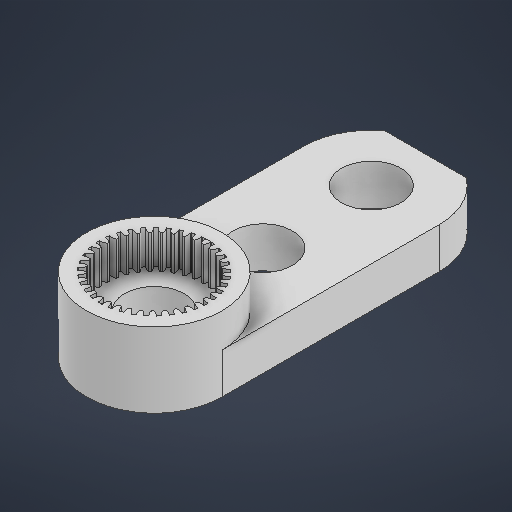
# Autodesk Inventor part: digital servo cap
Saved by Autodesk Inventor 2026.1 (Build 301233020, 233B)
## iProperties
Created: 2025-11-05
Part Number: digital servo cap
Material: Generic
Document SubType Name: Modeling
Designer: Asus
Density: 1 g/cm^3
Appearance: Default
Author: Asus
Autodesk Inventor part; units mm, degrees
ref_plane "YZ Plane" through (0, 0, 0) normal (1, 0, 0) x (0, 1, 0)
ref_plane "XZ Plane" through (0, 0, 0) normal (0, 1, 0) x (-1, 0, 0)
ref_plane "XY Plane" through (0, 0, 0) normal (0, 0, 1) x (1, 0, 0)
sketch "Sketch1" plane through (0, 0, 0) normal (0, 1, 0) x (-1, 0, 0)
  line L0 (0, 0) -> (0, -16) construction
  line L1 (-5, 0) -> (-5, -16)
  line L2 (5, -16) -> (5, 0)
  arc A0 (5, 0) -> (-5, 0) centre (0, 0) ccw
  circle A1 centre (0, 0) radius 2.2
  circle A2 centre (0, -16) radius 2.2
  line L3 (0, -16) -> (0, -20)
  line L4 (0, -20) -> (3, -20)
  line L5 (3, -20) -> (-3, -20)
  arc A3 (-5, -16) -> (-3, -20) centre (0, -16) ccw
  arc A4 (3, -20) -> (5, -16) centre (0, -16) ccw
  circle A5 centre (0, -8) radius 2.2
  dimension "d0" = 16
  dimension "d2" = 4.4
  dimension "d3" = 4.4
  dimension "d4" = 4
  dimension "d5" = 4.4
  constraints: 14 end point, 6 centre point, 6 point on circle, 4 tangent, 3 coincident, 2 vertical, 1 midpoint, 1 parallel, 1 perpendicular
  measures "d0" distance of L0.start L0.end
  measures "d2" diameter of A1
  measures "d3" diameter of A2
  measures "d4" distance of L3.start L3.end
  measures "d5" diameter of A5
extrude "Extrusion1" add sketch "Sketch1" along normal blind 3
sketch "Sketch2" plane through (0, 3, 0) normal (0, 1, 0) x (1, 0, 0)
  circle A0 centre (0, 0) radius 4
  circle A1 centre (0, 0) radius 5
  dimension "d8" = 8
  constraints: 2 centre point, 2 coincident
  measures "d8" diameter of A0
extrude "Extrusion2" add sketch "Sketch2" along normal blind 2.5
sketch "Sketch3" plane through (0, 5.5, 0) normal (0, 1, 0) x (1, 0, 0)
  circle A0 centre (0, 0) radius 4
  circle A1 centre (0, 0) radius 4 projected
  line L0 (0, 4.0912) -> (0, 3.5243) construction
  line L1 (-0.2, 3.995) -> (0.2, 3.995)
  circle A2 centre (0, 0) radius 4 projected
  line L2 (0, 3.545) -> (0.075, 3.545)
  line L3 (0, 3.545) -> (-0.075, 3.545)
  arc A3 (-0.1998, 3.9692) -> (-0.075, 3.545) centre (0.65, 3.9887) ccw
  arc A4 (0.075, 3.545) -> (0.1998, 3.9692) centre (-0.65, 3.9887) ccw
  arc A5 (0.2262, 3.9936) -> (0.1998, 3.9692) centre (0.2248, 3.9686) ccw
  arc A6 (-0.1998, 3.9692) -> (-0.2262, 3.9936) centre (-0.2248, 3.9686) ccw
  line L4 (-0.5991, 3.494) -> (-0.673, 3.4813)
  line L5 (-0.5991, 3.494) -> (-0.5252, 3.5067)
  arc A7 (-0.5252, 3.5067) -> (-0.4739, 3.9459) centre (-1.3147, 3.8215) ccw
  arc A8 (-0.8677, 3.8784) -> (-0.673, 3.4813) centre (-0.0335, 4.0412) ccw
  arc A9 (-0.8677, 3.8784) -> (-0.8979, 3.8979) centre (-0.8923, 3.8736) ccw
  arc A10 (-0.452, 3.9744) -> (-0.4739, 3.9459) centre (-0.4491, 3.9495) ccw
  line L6 (-1.181, 3.3425) -> (-1.2517, 3.3175)
  line L7 (-1.181, 3.3425) -> (-1.1103, 3.3675)
  arc A11 (-1.1103, 3.3675) -> (-1.1339, 3.809) centre (-1.9417, 3.5444) ccw
  arc A12 (-1.5107, 3.6759) -> (-1.2517, 3.3175) centre (-0.716, 3.9774) ccw
  arc A13 (-1.5107, 3.6759) -> (-1.5437, 3.6901) centre (-1.5341, 3.6671) ccw
  arc A14 (-1.1171, 3.8408) -> (-1.1339, 3.809) centre (-1.1102, 3.8168) ccw
  line L8 (-1.7289, 3.0948) -> (-1.7944, 3.0583)
  line L9 (-1.7289, 3.0948) -> (-1.6634, 3.1314)
  arc A15 (-1.6634, 3.1314) -> (-1.7613, 3.5626) centre (-2.5127, 3.1652) ccw
  arc A16 (-2.1102, 3.3677) -> (-1.7944, 3.0583) centre (-1.3778, 3.7992) ccw
  arc A17 (-2.1102, 3.3677) -> (-2.1451, 3.3761) centre (-2.1317, 3.355) ccw
  arc A18 (-1.7502, 3.5968) -> (-1.7613, 3.5626) centre (-1.7392, 3.5743) ccw
  line L10 (-2.227, 2.7581) -> (-2.2854, 2.711)
  line L11 (-2.227, 2.7581) -> (-2.1687, 2.8053)
  arc A19 (-2.1687, 2.8053) -> (-2.3381, 3.2137) centre (-3.0115, 2.6951) ccw
  arc A20 (-2.649, 2.9627) -> (-2.2854, 2.711) centre (-2.0001, 3.5117) ccw
  arc A21 (-2.649, 2.9627) -> (-2.6849, 2.9651) centre (-2.6681, 2.9465) ccw
  arc A22 (-2.3329, 3.2493) -> (-2.3381, 3.2137) centre (-2.3183, 3.229) ccw
  line L12 (-2.6611, 2.3421) -> (-2.7107, 2.2858)
  line L13 (-2.6611, 2.3421) -> (-2.6116, 2.3984)
  arc A23 (-2.6116, 2.3984) -> (-2.8476, 2.7723) centre (-3.4237, 2.1473) ccw
  arc A24 (-3.1116, 2.4724) -> (-2.7107, 2.2858) centre (-2.5648, 3.1232) ccw
  arc A25 (-3.1116, 2.4724) -> (-3.1473, 2.4687) centre (-3.1277, 2.4532) ccw
  arc A26 (-2.8484, 2.8083) -> (-2.8476, 2.7723) centre (-2.8306, 2.7907) ccw
  line L14 (-3.0187, 1.8587) -> (-3.058, 1.7948)
  line L15 (-3.0187, 1.8587) -> (-2.9793, 1.9225)
  arc A27 (-2.9793, 1.9225) -> (-3.2751, 2.2512) centre (-3.7373, 1.5379) ccw
  arc A28 (-3.4847, 1.911) -> (-3.058, 1.7948) centre (-3.0557, 2.6448) ccw
  arc A29 (-3.4847, 1.911) -> (-3.5193, 1.9013) centre (-3.4973, 1.8894) ccw
  arc A30 (-3.2821, 2.2865) -> (-3.2751, 2.2512) centre (-3.2616, 2.2722) ccw
  line L16 (-3.2894, 1.3218) -> (-3.3173, 1.2522)
  line L17 (-3.2894, 1.3218) -> (-3.2614, 1.3914)
  arc A31 (-3.2614, 1.3914) -> (-3.6085, 1.6653) centre (-3.9435, 0.8841) ccw
  arc A32 (-3.7575, 1.2946) -> (-3.3173, 1.2522) centre (-3.4588, 2.0903) ccw
  arc A33 (-3.7575, 1.2946) -> (-3.79, 1.2791) centre (-3.7663, 1.2712) ccw
  arc A34 (-3.6213, 1.6989) -> (-3.6085, 1.6653) centre (-3.5986, 1.6883) ccw
  line L18 (-3.4654, 0.7469) -> (-3.4812, 0.6735)
  line L19 (-3.4654, 0.7469) -> (-3.4496, 0.8202)
  arc A35 (-3.4496, 0.8202) -> (-3.838, 1.0315) centre (-4.0362, 0.205) ccw
  arc A36 (-3.9222, 0.6409) -> (-3.4812, 0.6735) centre (-3.7623, 1.4757) ccw
  arc A37 (-3.9222, 0.6409) -> (-3.9516, 0.6202) centre (-3.9269, 0.6164) ccw
  arc A38 (-3.8563, 1.0625) -> (-3.838, 1.0315) centre (-3.8322, 1.0559) ccw
  line L20 (-3.5418, 0.1505) -> (-3.545, 0.0755)
  line L21 (-3.5418, 0.1505) -> (-3.5386, 0.2254)
  arc A39 (-3.5386, 0.2254) -> (-3.9572, 0.3681) centre (-4.0127, -0.4801) ccw
  arc A40 (-3.9741, -0.0312) -> (-3.545, 0.0755) centre (-3.9576, 0.8187) ccw
  arc A41 (-3.9741, -0.0312) -> (-3.9996, -0.0565) centre (-3.9746, -0.0562) ccw
  arc A42 (-3.9804, 0.3955) -> (-3.9572, 0.3681) centre (-3.9555, 0.393) ccw
  line L22 (-3.5163, -0.4503) -> (-3.5068, -0.5247)
  line L23 (-3.5163, -0.4503) -> (-3.5258, -0.3759)
  arc A43 (-3.5258, -0.3759) -> (-3.9624, -0.306) centre (-3.8739, -1.1514) ccw
  arc A44 (-3.9117, -0.7023) -> (-3.5068, -0.5247) centre (-4.039, 0.1381) ccw
  arc A45 (-3.9117, -0.7023) -> (-3.9325, -0.7316) centre (-3.9079, -0.7271) ccw
  arc A46 (-3.99, -0.2829) -> (-3.9624, -0.306) centre (-3.965, -0.2811) ccw
  line L24 (-3.3896, -1.0381) -> (-3.3676, -1.1098)
  line L25 (-3.3896, -1.0381) -> (-3.4116, -0.9663)
  arc A47 (-3.4116, -0.9663) -> (-3.8537, -0.9712) centre (-3.6236, -1.7895) ccw
  arc A48 (-3.7367, -1.3533) -> (-3.3676, -1.1098) centre (-4.0042, -0.5465) ccw
  arc A49 (-3.7367, -1.3533) -> (-3.7523, -1.3857) centre (-3.7289, -1.377) ccw
  arc A50 (-3.8848, -0.9531) -> (-3.8537, -0.9712) centre (-3.8605, -0.9472) ccw
  line L26 (-3.1654, -1.596) -> (-3.1317, -1.6629)
  line L27 (-3.1654, -1.596) -> (-3.1992, -1.529)
  arc A51 (-3.1992, -1.529) -> (-3.6342, -1.6085) centre (-3.269, -2.3761) ccw
  arc A52 (-3.4543, -1.9654) -> (-3.1317, -1.6629) centre (-3.8543, -1.2154) ccw
  arc A53 (-3.4543, -1.9654) -> (-3.4641, -1.9999) centre (-3.4425, -1.9874) ccw
  arc A54 (-3.6678, -1.5959) -> (-3.6342, -1.6085) centre (-3.6449, -1.586) ccw
  line L28 (-2.8502, -2.108) -> (-2.8056, -2.1683)
  line L29 (-2.8502, -2.108) -> (-2.8948, -2.0477)
  arc A55 (-2.8948, -2.0477) -> (-3.31, -2.1996) centre (-2.8204, -2.8944) ccw
  arc A56 (-3.0724, -2.5209) -> (-2.8056, -2.1683) centre (-3.5934, -1.8493) ccw
  arc A57 (-3.0724, -2.5209) -> (-3.0763, -2.5566) centre (-3.0571, -2.5406) ccw
  arc A58 (-3.3454, -2.1929) -> (-3.31, -2.1996) centre (-3.3244, -2.1792) ccw
  line L30 (-2.4529, -2.5593) -> (-2.3988, -2.6112)
  line L31 (-2.4529, -2.5593) -> (-2.5071, -2.5074)
  arc A59 (-2.5071, -2.5074) -> (-2.8907, -2.7273) centre (-2.2907, -3.3294) ccw
  arc A60 (-2.6022, -3.0038) -> (-2.3988, -2.6112) centre (-3.2292, -2.43) ccw
  arc A61 (-2.6022, -3.0038) -> (-2.6, -3.0397) centre (-2.5838, -3.0207) ccw
  arc A62 (-2.9266, -2.7267) -> (-2.8907, -2.7273) centre (-2.9083, -2.7096) ccw
  line L32 (-1.9851, -2.9371) -> (-1.923, -2.9791)
  line L33 (-1.9851, -2.9371) -> (-2.0472, -2.8951)
  arc A63 (-2.0472, -2.8951) -> (-2.3882, -3.1766) centre (-1.6951, -3.6687) ccw
  arc A64 (-2.0571, -3.4004) -> (-1.923, -2.9791) centre (-2.7721, -2.9407) ccw
  arc A65 (-2.0571, -3.4004) -> (-2.0489, -3.4354) centre (-2.0361, -3.4139) ccw
  arc A66 (-2.4237, -3.1821) -> (-2.3882, -3.1766) centre (-2.4086, -3.1622) ccw
  line L34 (-1.4602, -3.2303) -> (-1.3918, -3.2612)
  line L35 (-1.4602, -3.2303) -> (-1.5285, -3.1994)
  arc A67 (-1.5285, -3.1994) -> (-1.817, -3.5346) centre (-1.0507, -3.9024) ccw
  arc A68 (-1.4529, -3.6992) -> (-1.3918, -3.2612) centre (-2.2352, -3.3669) ccw
  arc A69 (-1.4529, -3.6992) -> (-1.4388, -3.7323) centre (-1.4299, -3.7089) ccw
  arc A70 (-1.8511, -3.5459) -> (-1.817, -3.5346) centre (-1.8395, -3.5237) ccw
  line L36 (-0.8933, -3.4306) -> (-0.8207, -3.4495)
  line L37 (-0.8933, -3.4306) -> (-0.9658, -3.4117)
  arc A71 (-0.9658, -3.4117) -> (-1.1935, -3.7908) centre (-0.3761, -4.0238) ccw
  arc A72 (-0.8068, -3.8915) -> (-0.8207, -3.4495) centre (-1.6341, -3.6963) ccw
  arc A73 (-0.8068, -3.8915) -> (-0.7874, -3.9217) centre (-0.7825, -3.8972) ccw
  arc A74 (-1.2252, -3.8077) -> (-1.1935, -3.7908) centre (-1.2175, -3.7839) ccw
  line L38 (-0.3006, -3.5322) -> (-0.2259, -3.5386)
  line L39 (-0.3006, -3.5322) -> (-0.3754, -3.5259)
  arc A75 (-0.3754, -3.5259) -> (-0.5357, -3.938) centre (0.3094, -4.0295) ccw
  arc A76 (-0.1375, -3.9719) -> (-0.2259, -3.5386) centre (-0.9859, -3.9192) ccw
  arc A77 (-0.1375, -3.9719) -> (-0.1133, -3.9984) centre (-0.1126, -3.9734) ccw
  arc A78 (-0.5641, -3.96) -> (-0.5357, -3.938) centre (-0.5605, -3.9353) ccw
  line L40 (0.3006, -3.5322) -> (0.3754, -3.5259)
  line L41 (0.3006, -3.5322) -> (0.2259, -3.5386)
  arc A79 (0.2259, -3.5386) -> (0.1375, -3.9719) centre (0.9859, -3.9192) ccw
  arc A80 (0.5357, -3.938) -> (0.3754, -3.5259) centre (-0.3094, -4.0295) ccw
  arc A81 (0.5357, -3.938) -> (0.5641, -3.96) centre (0.5605, -3.9353) ccw
  arc A82 (0.1133, -3.9984) -> (0.1375, -3.9719) centre (0.1126, -3.9734) ccw
  line L42 (0.8933, -3.4306) -> (0.9658, -3.4117)
  line L43 (0.8933, -3.4306) -> (0.8207, -3.4495)
  arc A83 (0.8207, -3.4495) -> (0.8068, -3.8915) centre (1.6341, -3.6963) ccw
  arc A84 (1.1935, -3.7908) -> (0.9658, -3.4117) centre (0.3761, -4.0238) ccw
  arc A85 (1.1935, -3.7908) -> (1.2252, -3.8077) centre (1.2175, -3.7839) ccw
  arc A86 (0.7874, -3.9217) -> (0.8068, -3.8915) centre (0.7825, -3.8972) ccw
  line L44 (1.4602, -3.2303) -> (1.5285, -3.1994)
  line L45 (1.4602, -3.2303) -> (1.3918, -3.2612)
  arc A87 (1.3918, -3.2612) -> (1.4529, -3.6992) centre (2.2352, -3.3669) ccw
  arc A88 (1.817, -3.5346) -> (1.5285, -3.1994) centre (1.0507, -3.9024) ccw
  arc A89 (1.817, -3.5346) -> (1.8511, -3.5459) centre (1.8395, -3.5237) ccw
  arc A90 (1.4388, -3.7323) -> (1.4529, -3.6992) centre (1.4299, -3.7089) ccw
  line L46 (1.9851, -2.9371) -> (2.0472, -2.8951)
  line L47 (1.9851, -2.9371) -> (1.923, -2.9791)
  arc A91 (1.923, -2.9791) -> (2.0571, -3.4004) centre (2.7721, -2.9407) ccw
  arc A92 (2.3882, -3.1766) -> (2.0472, -2.8951) centre (1.6951, -3.6687) ccw
  arc A93 (2.3882, -3.1766) -> (2.4237, -3.1821) centre (2.4086, -3.1622) ccw
  arc A94 (2.0489, -3.4354) -> (2.0571, -3.4004) centre (2.0361, -3.4139) ccw
  line L48 (2.4529, -2.5593) -> (2.5071, -2.5074)
  line L49 (2.4529, -2.5593) -> (2.3988, -2.6112)
  arc A95 (2.3988, -2.6112) -> (2.6022, -3.0038) centre (3.2292, -2.43) ccw
  arc A96 (2.8907, -2.7273) -> (2.5071, -2.5074) centre (2.2907, -3.3294) ccw
  arc A97 (2.8907, -2.7273) -> (2.9266, -2.7267) centre (2.9083, -2.7096) ccw
  arc A98 (2.6, -3.0397) -> (2.6022, -3.0038) centre (2.5838, -3.0207) ccw
  line L50 (2.8502, -2.108) -> (2.8948, -2.0477)
  line L51 (2.8502, -2.108) -> (2.8056, -2.1683)
  arc A99 (2.8056, -2.1683) -> (3.0724, -2.5209) centre (3.5934, -1.8493) ccw
  arc A100 (3.31, -2.1996) -> (2.8948, -2.0477) centre (2.8204, -2.8944) ccw
  arc A101 (3.31, -2.1996) -> (3.3454, -2.1929) centre (3.3244, -2.1792) ccw
  arc A102 (3.0763, -2.5566) -> (3.0724, -2.5209) centre (3.0571, -2.5406) ccw
  line L52 (3.1654, -1.596) -> (3.1992, -1.529)
  line L53 (3.1654, -1.596) -> (3.1317, -1.6629)
  arc A103 (3.1317, -1.6629) -> (3.4543, -1.9654) centre (3.8543, -1.2154) ccw
  arc A104 (3.6342, -1.6085) -> (3.1992, -1.529) centre (3.269, -2.3761) ccw
  arc A105 (3.6342, -1.6085) -> (3.6678, -1.5959) centre (3.6449, -1.586) ccw
  arc A106 (3.4641, -1.9999) -> (3.4543, -1.9654) centre (3.4425, -1.9874) ccw
  line L54 (3.3896, -1.0381) -> (3.4116, -0.9663)
  line L55 (3.3896, -1.0381) -> (3.3676, -1.1098)
  arc A107 (3.3676, -1.1098) -> (3.7367, -1.3533) centre (4.0042, -0.5465) ccw
  arc A108 (3.8537, -0.9712) -> (3.4116, -0.9663) centre (3.6236, -1.7895) ccw
  arc A109 (3.8537, -0.9712) -> (3.8848, -0.9531) centre (3.8605, -0.9472) ccw
  arc A110 (3.7523, -1.3857) -> (3.7367, -1.3533) centre (3.7289, -1.377) ccw
  line L56 (3.5163, -0.4503) -> (3.5258, -0.3759)
  line L57 (3.5163, -0.4503) -> (3.5068, -0.5247)
  arc A111 (3.5068, -0.5247) -> (3.9117, -0.7023) centre (4.039, 0.1381) ccw
  arc A112 (3.9624, -0.306) -> (3.5258, -0.3759) centre (3.8739, -1.1514) ccw
  arc A113 (3.9624, -0.306) -> (3.99, -0.2829) centre (3.965, -0.2811) ccw
  arc A114 (3.9325, -0.7316) -> (3.9117, -0.7023) centre (3.9079, -0.7271) ccw
  line L58 (3.5418, 0.1505) -> (3.5386, 0.2254)
  line L59 (3.5418, 0.1505) -> (3.545, 0.0755)
  arc A115 (3.545, 0.0755) -> (3.9741, -0.0312) centre (3.9576, 0.8187) ccw
  arc A116 (3.9572, 0.3681) -> (3.5386, 0.2254) centre (4.0127, -0.4801) ccw
  arc A117 (3.9572, 0.3681) -> (3.9804, 0.3955) centre (3.9555, 0.393) ccw
  arc A118 (3.9996, -0.0565) -> (3.9741, -0.0312) centre (3.9746, -0.0562) ccw
  line L60 (3.4654, 0.7469) -> (3.4496, 0.8202)
  line L61 (3.4654, 0.7469) -> (3.4812, 0.6735)
  arc A119 (3.4812, 0.6735) -> (3.9222, 0.6409) centre (3.7623, 1.4757) ccw
  arc A120 (3.838, 1.0315) -> (3.4496, 0.8202) centre (4.0362, 0.205) ccw
  arc A121 (3.838, 1.0315) -> (3.8563, 1.0625) centre (3.8322, 1.0559) ccw
  arc A122 (3.9516, 0.6202) -> (3.9222, 0.6409) centre (3.9269, 0.6164) ccw
  line L62 (3.2894, 1.3218) -> (3.2614, 1.3914)
  line L63 (3.2894, 1.3218) -> (3.3173, 1.2522)
  arc A123 (3.3173, 1.2522) -> (3.7575, 1.2946) centre (3.4588, 2.0903) ccw
  arc A124 (3.6085, 1.6653) -> (3.2614, 1.3914) centre (3.9435, 0.8841) ccw
  arc A125 (3.6085, 1.6653) -> (3.6213, 1.6989) centre (3.5986, 1.6883) ccw
  arc A126 (3.79, 1.2791) -> (3.7575, 1.2946) centre (3.7663, 1.2712) ccw
  line L64 (3.0187, 1.8587) -> (2.9793, 1.9225)
  line L65 (3.0187, 1.8587) -> (3.058, 1.7948)
  arc A127 (3.058, 1.7948) -> (3.4847, 1.911) centre (3.0557, 2.6448) ccw
  arc A128 (3.2751, 2.2512) -> (2.9793, 1.9225) centre (3.7373, 1.5379) ccw
  arc A129 (3.2751, 2.2512) -> (3.2821, 2.2865) centre (3.2616, 2.2722) ccw
  arc A130 (3.5193, 1.9013) -> (3.4847, 1.911) centre (3.4973, 1.8894) ccw
  line L66 (2.6611, 2.3421) -> (2.6116, 2.3984)
  line L67 (2.6611, 2.3421) -> (2.7107, 2.2858)
  arc A131 (2.7107, 2.2858) -> (3.1116, 2.4724) centre (2.5648, 3.1232) ccw
  arc A132 (2.8476, 2.7723) -> (2.6116, 2.3984) centre (3.4237, 2.1473) ccw
  arc A133 (2.8476, 2.7723) -> (2.8484, 2.8083) centre (2.8306, 2.7907) ccw
  arc A134 (3.1473, 2.4687) -> (3.1116, 2.4724) centre (3.1277, 2.4532) ccw
  line L68 (2.227, 2.7581) -> (2.1687, 2.8053)
  line L69 (2.227, 2.7581) -> (2.2854, 2.711)
  arc A135 (2.2854, 2.711) -> (2.649, 2.9627) centre (2.0001, 3.5117) ccw
  arc A136 (2.3381, 3.2137) -> (2.1687, 2.8053) centre (3.0115, 2.6951) ccw
  arc A137 (2.3381, 3.2137) -> (2.3329, 3.2493) centre (2.3183, 3.229) ccw
  arc A138 (2.6849, 2.9651) -> (2.649, 2.9627) centre (2.6681, 2.9465) ccw
  line L70 (1.7289, 3.0948) -> (1.6634, 3.1314)
  line L71 (1.7289, 3.0948) -> (1.7944, 3.0583)
  arc A139 (1.7944, 3.0583) -> (2.1102, 3.3677) centre (1.3778, 3.7992) ccw
  arc A140 (1.7613, 3.5626) -> (1.6634, 3.1314) centre (2.5127, 3.1652) ccw
  arc A141 (1.7613, 3.5626) -> (1.7502, 3.5968) centre (1.7392, 3.5743) ccw
  arc A142 (2.1451, 3.3761) -> (2.1102, 3.3677) centre (2.1317, 3.355) ccw
  line L72 (1.181, 3.3425) -> (1.1103, 3.3675)
  line L73 (1.181, 3.3425) -> (1.2517, 3.3175)
  arc A143 (1.2517, 3.3175) -> (1.5107, 3.6759) centre (0.716, 3.9774) ccw
  arc A144 (1.1339, 3.809) -> (1.1103, 3.3675) centre (1.9417, 3.5444) ccw
  arc A145 (1.1339, 3.809) -> (1.1171, 3.8408) centre (1.1102, 3.8168) ccw
  arc A146 (1.5437, 3.6901) -> (1.5107, 3.6759) centre (1.5341, 3.6671) ccw
  line L74 (0.5991, 3.494) -> (0.5252, 3.5067)
  line L75 (0.5991, 3.494) -> (0.673, 3.4813)
  arc A147 (0.673, 3.4813) -> (0.8677, 3.8784) centre (0.0335, 4.0412) ccw
  arc A148 (0.4739, 3.9459) -> (0.5252, 3.5067) centre (1.3147, 3.8215) ccw
  arc A149 (0.4739, 3.9459) -> (0.452, 3.9744) centre (0.4491, 3.9495) ccw
  arc A150 (0.8979, 3.8979) -> (0.8677, 3.8784) centre (0.8923, 3.8736) ccw
  circle A151 centre (0, 0) radius 4
  point P0 (0.452, 3.9744)
  point P1 (1.5437, 3.6901)
  point P2 (3.1473, 2.4687)
  point P3 (2.8484, 2.8083)
  point P4 (3.79, 1.2791)
  point P5 (3.6213, 1.6989)
  point P6 (3.8563, 1.0625)
  point P7 (3.99, -0.2829)
  point P8 (3.7523, -1.3857)
  point P9 (3.8848, -0.9531)
  point P10 (3.4641, -1.9999)
  point P11 (0.1133, -3.9984)
  point P12 (-0.5641, -3.96)
  point P13 (-0.1133, -3.9984)
  point P14 (-1.2252, -3.8077)
  point P15 (-0.7874, -3.9217)
  point P16 (-2.0489, -3.4354)
  point P17 (-2.9266, -2.7267)
  point P18 (-2.6, -3.0397)
  point P19 (-3.0763, -2.5566)
  point P20 (-3.8848, -0.9531)
  point P21 (-3.99, -0.2829)
  point P22 (-3.9996, -0.0565)
  point P23 (-3.79, 1.2791)
  point P24 (-2.1451, 3.3761)
  point P25 (-0.2262, 3.9936)
  dimension "d15" = 0.4
  dimension "d17" = 0.075
  dimension "d18" = 0.075
  dimension "d19" = 0.85
  dimension "d20" = 0.85
  dimension "d21" = 0.05
  dimension "d22" = 0.05
  dimension "d25" = 360
  constraints: 300 point on circle, 152 end point, 148 centre point, 4 tangent, 2 coincident, 2 horizontal, 1 perpendicular, 1 point on line, 1 vertical, 634 other
  measures "d15" distance of L1.start L1.end
  measures "d17" distance of L2.start L2.end
  measures "d18" distance of L2.start L3.end
  measures "d19" radius of A3
  measures "d20" radius of A4
  measures "d21" diameter of A5
  measures "d22" diameter of A6
extrude "Extrusion3" add sketch "Sketch3" against normal blind 3 contours A0 A118 A115 L59 L58 A116 A117 | A122 A119 L61 L60 A120 A121 A0 | A0 A114 A111 L57 L56 A112 A113 | A126 A123 L63 L62 A124 A125 A0 | A0 A110 A107 L55 L54 A108 A109 | A130 A127 L65 L64 A128 A129 A0 | A0 A106 A103 L53 L52 A104 A105 | A134 A131 L67 L66 A132 A133 A0 | A0 A102 A99 L51 L50 A100 A101 | A138 A135 L69 L68 A136 A137 A0 | A0 A98 A95 L49 L48 A96 A97 | A142 A139 L71 L70 A140 A141 A0 | A0 A94 A91 L47 L46 A92 A93 | A146 A143 L73 L72 A144 A145 A0 | A0 A90 A87 L45 L44 A88 A89 | A150 A147 L75 L74 A148 A149 A0 | A0 A86 A83 L43 L42 A84 A85 | A5 A4 L2 L3 A3 A6 A0 L1 | A0 A82 A79 L41 L40 A80 A81 | A0 A78 A75 L39 L38 A76 A77 | A10 A7 L5 L4 A8 A9 A0 | A0 A74 A71 L37 L36 A72 A73 | A14 A11 L7 L6 A12 A13 A0 | A0 A70 A67 L35 L34 A68 A69 | A18 A15 L9 L8 A16 A17 A0 | A0 A66 A63 L33 L32 A64 A65 | A22 A19 L11 L10 A20 A21 A0 | A0 A62 A59 L31 L30 A60 A61 | A26 A23 L13 L12 A24 A25 A0 | A0 A58 A55 L29 L28 A56 A57 | A30 A27 L15 L14 A28 A29 A0 | A0 A54 A51 L27 L26 A52 A53 | A34 A31 L17 L16 A32 A33 A0 | A0 A50 A47 L25 L24 A48 A49 | A38 A35 L19 L18 A36 A37 A0 | A0 A46 A43 L23 L22 A44 A45 | A42 A39 L21 L20 A40 A41 A0
body "Solid1"
